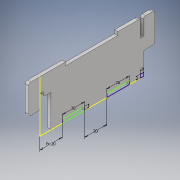
# Autodesk Inventor part: cham_right_v2
Saved by Autodesk Inventor 2017.2 (Build 212233000, 233)
## iProperties
Created: 2017-06-09
Part Number: cham_right_v2
Material: Generic
Document SubType Name: Modeling
Designer: SandeepSH
Density: 1 g/cm^3
Appearance: Default
Author: SandeepSH
Autodesk Inventor part; units mm, degrees
ref_plane "YZ Plane" through (0, 0, 0) normal (1, 0, 0) x (0, 1, 0)
ref_plane "XZ Plane" through (0, 0, 0) normal (0, 1, 0) x (-1, 0, 0)
ref_plane "XY Plane" through (0, 0, 0) normal (0, 0, 1) x (1, 0, 0)
sketch "Sketch1" plane through (0, 0, 0) normal (1, 0, 0) x (0, 1, 0)
  line L0 (0, 0) -> (46, 0)
  line L1 (46, 0) -> (46, -93)
  line L2 (46, -93) -> (0, -93)
  line L3 (0, -93) -> (0, 0)
  dimension "d0" = 46
  dimension "d1" = 93
  constraints: 8 end point, 2 parallel, 1 horizontal, 1 perpendicular
  measures "d0" distance of L1.end L2.end
  measures "d1" distance of L0.end L1.end
extrude "Extrusion1" add sketch "Sketch1" along normal blind 3
sketch "Sketch2" plane through (3, 0, 0) normal (1, 0, 0) x (0, 0, -1)
  line L0 (20, 0) -> (40, 0)
  line L1 (40, 0) -> (40, 3)
  line L2 (40, 3) -> (20, 3)
  line L3 (20, 3) -> (20, 0)
  line L4 (0, 46) -> (0, 0) projected
  line L5 (0, 0) -> (93, 0) projected
  line L6 (60, 0) -> (80, 0)
  line L7 (80, 0) -> (80, 3)
  line L8 (80, 3) -> (60, 3)
  line L9 (60, 3) -> (60, 0)
  line L10 (93, 0) -> (90, 0)
  line L11 (90, 0) -> (90, 3)
  line L12 (90, 3) -> (93, 3)
  line L13 (93, 3) -> (93, 0)
  dimension "d4" = 20
  dimension "d5" = 3
  dimension "d6" = 20
  dimension "d7" = 20
  dimension "d8" = 20
  dimension "d11" = 3
  dimension "d12" = 3
  constraints: 24 end point, 6 parallel, 3 horizontal, 3 perpendicular, 1 point on line
  measures "d4" distance of L2.end L1.end
  measures "d5" distance of L1.end L0.end
  measures "d6" distance between parallel lines of L3 L4
  measures "d7" distance of L8.end L7.end
  measures "d8" distance between parallel lines of L9 L1
  measures "d11" distance of L11.end L12.end
  measures "d12" distance of L10.end L11.end
extrude "Extrusion2" cut sketch "Sketch2" against normal through all contours L3 L2 L1 L0 | L9 L8 L7 L5
extrude "Extrusion3" cut sketch "Sketch2" against normal through all contours L11 L12 L13 L5
sketch "Sketch3" plane through (3, 0, 0) normal (1, 0, 0) x (0, 0, -1)
  point P0 (0, 0)
sketch "Sketch4" plane through (3, 0, 0) normal (1, 0, 0) x (0, 0, -1)
  point P0 (0, 0)
sketch "Sketch5" plane through (3, 0, 0) normal (1, 0, 0) x (0, 0, -1)
  line L0 (0, 0) -> (0, 46) projected
  line L1 (0, 46) -> (-10, 46)
  line L2 (-10, 46) -> (-10, 20)
  line L3 (-10, 20) -> (0, 20)
  line L4 (0, 20) -> (0, 46)
  line L5 (0, 0) -> (20, 0) projected
  line L6 (93, 46) -> (103, 46)
  line L7 (103, 46) -> (103, 20)
  line L8 (103, 20) -> (93, 20)
  line L9 (93, 20) -> (93, 46)
  dimension "d15" = 10
  dimension "d16" = 20
  dimension "d28" = 10
  dimension "d29" = 20
  constraints: 16 end point, 4 parallel, 2 horizontal, 2 perpendicular
  measures "d15" distance of L3.end L2.end
  measures "d16" distance between parallel lines of L5 L3
  measures "d28" distance between parallel lines of L7 L9
  measures "d29" distance between parallel lines of L5 L8
extrude "Extrusion6" add sketch "Sketch5" against normal blind 3 contours L6 L7 L8 L9
fillet "Fillet1" radius 2 3 edges at (1.5, 46, -103) (1.5, 20, -103) (1.5, 20, -93) curvature continuous yes
sketch "Sketch7" plane through (3, 0, 0) normal (1, 0, 0) x (0, 0, -1)
  point P0 (0, 0)
sketch "Sketch8" plane through (3, 0, 0) normal (1, 0, 0) x (0, 0, -1)
  line L0 (0, 46) -> (0, 0) projected
  line L1 (0, 0) -> (10, 0)
  line L2 (10, 0) -> (10, 29)
  line L3 (10, 29) -> (0, 29)
  line L4 (0, 29) -> (0, 0)
  dimension "d33" = 10
  dimension "d34" = 29
  constraints: 8 end point, 2 parallel, 1 horizontal, 1 perpendicular
  measures "d33" distance of L3.end L2.end
  measures "d34" distance of L2.end L1.end
extrude "Extrusion7" cut sketch "Sketch8" against normal through all
sketch "Sketch9" plane through (3, 0, 0) normal (1, 0, 0) x (0, 0, -1)
  line L0 (0, 46) -> (101, 46) projected
  line L1 (0, 46) -> (-10, 46)
  line L2 (-10, 46) -> (-10, 20)
  line L3 (-10, 20) -> (0, 20)
  line L4 (0, 20) -> (0, 46)
  line L5 (10, 0) -> (20, 0) projected
  point P0 (0, 0)
  dimension "d37" = 10
  dimension "d39" = 20
  constraints: 8 end point, 2 parallel, 1 horizontal, 1 perpendicular
  measures "d37" distance of L3.end L2.end
  measures "d39" distance between parallel lines of L5 L3
extrude "Extrusion8" add sketch "Sketch9" against normal blind 3
sketch "Sketch10" plane through (3, 0, 0) normal (1, 0, 0) x (0, 0, -1)
  line L0 (0, 29) -> (0, 20) projected
  line L1 (0, 29) -> (3, 29)
  line L2 (3, 29) -> (3, 33)
  line L3 (3, 33) -> (0, 33)
  line L4 (0, 33) -> (0, 29)
  point P0 (0, 0)
  dimension "d42" = 3
  dimension "d43" = 4
  constraints: 8 end point, 2 parallel, 1 horizontal, 1 perpendicular
  measures "d42" distance of L3.end L2.end
  measures "d43" distance of L2.end L1.end
extrude "Extrusion9" cut sketch "Sketch10" against normal through all
fillet "Fillet2" radius 2 4 edges at (1.5, 20, 10) (1.5, 20, 0) (1.5, 29, -3) (1.5, 46, 10) curvature continuous yes
sketch "Sketch11" plane through (3, 0, 0) normal (1, 0, 0) x (0, 0, -1)
  line L0 (-8, 46) -> (101, 46) projected
  line L1 (90, 46) -> (93, 46)
  line L2 (93, 46) -> (93, 31)
  line L3 (93, 31) -> (90, 31)
  line L4 (90, 31) -> (90, 46)
  line L5 (103, 44) -> (103, 22) projected
  point P0 (0, 0)
  dimension "d47" = 3
  dimension "d48" = 15
  dimension "d49" = 10
  constraints: 8 end point, 2 parallel, 1 horizontal, 1 perpendicular, 1 point on line
  measures "d47" distance of L2.end L3.end
  measures "d48" distance of L1.end L2.end
  measures "d49" distance between parallel lines of L5 L2
extrude "Extrusion10" cut sketch "Sketch11" against normal through all
fillet "Fillet3" radius 2 2 edges at (1.5, 46, -90) (1.5, 46, -93) curvature continuous yes
sketch "Sketch12" plane through (3, 0, 0) normal (1, 0, 0) x (0, 0, -1)
  line L0 (-8, 46) -> (88, 46) projected
  line L1 (23, 46) -> (70, 46)
  line L2 (70, 46) -> (70, 43)
  line L3 (70, 43) -> (23, 43)
  line L4 (23, 43) -> (23, 46)
  line L5 (90, 31) -> (90, 44) projected
  line L6 (3, 33) -> (3, 31) projected
  point P0 (0, 0)
  dimension "d53" = 3
  dimension "d54" = 20
  dimension "d55" = 20
  constraints: 8 end point, 2 parallel, 1 horizontal, 1 perpendicular, 1 point on line
  measures "d53" distance of L1.end L2.end
  measures "d54" distance between parallel lines of L5 L2
  measures "d55" distance between parallel lines of L4 L6
extrude "Extrusion11" cut sketch "Sketch12" against normal through all
equation "\"d6\" = d4"
equation "\"d28\" = d15"
equation "\"d29\" = d16"
body "Solid1"
